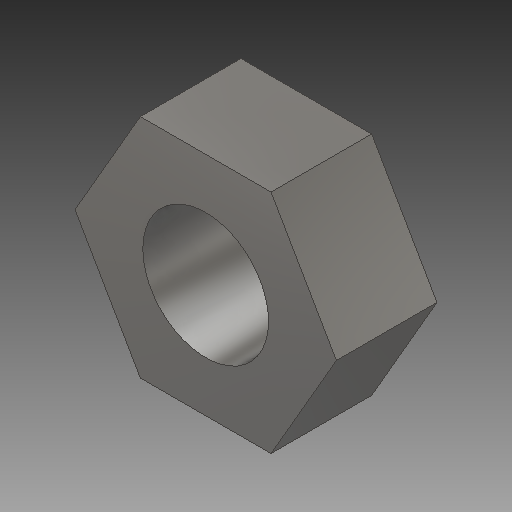
# Autodesk Inventor part: m3Nut
Saved by Autodesk Inventor 2019.4 (Build 234330000, 330)
## iProperties
Created: 2019-06-13
Part Number: m3Nut
Material: Stainless Steel
Document SubType Name: Modeling
Designer: mja502
Density: 8 g/cm^3
Appearance: Semi-Polished
m3Nut_diam: 5,400 mm
m3Nut_depth: 2,400 mm
Author: mja502
Autodesk Inventor part; units mm, degrees
ref_plane "YZ Plane" through (0, 0, 0) normal (1, 0, 0) x (0, 1, 0)
ref_plane "XZ Plane" through (0, 0, 0) normal (0, 1, 0) x (-1, 0, 0)
ref_plane "XY Plane" through (0, 0, 0) normal (0, 0, 1) x (1, 0, 0)
sketch "Sketch3" plane through (0, 0, 0) normal (0, 0, 1) x (1, 0, 0)
  line L0 (1.5588, -2.7) -> (-1.5588, -2.7)
  line L1 (-1.5588, -2.7) -> (-3.1177, 0)
  line L2 (-3.1177, 0) -> (-1.5588, 2.7)
  line L3 (-1.5588, 2.7) -> (1.5588, 2.7)
  line L4 (1.5588, 2.7) -> (3.1177, 0)
  line L5 (3.1177, 0) -> (1.5588, -2.7)
  circle A0 centre (0, 0) radius 1.5
  dimension "d12" = 5.4
  dimension "d13" = 3
  constraints: 12 end point, 2 coincident, 1 centre point, 1 horizontal, 13 other
  measures "d12" distance between parallel lines of L3 L0
  measures "d13" diameter of A0
extrude "Extrusion4" add sketch "Sketch3" along normal blind 2.4
equation "\"d12\" = m3Nut_diam"
equation "\"d14\" = m3Nut_depth"
equation "\"m3Nut_diam\" = 5.4"
equation "\"m3Nut_depth\" = 2.4"
body "Solid2"
